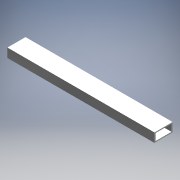
# Autodesk Inventor part: Extrusion Mid
Saved by Autodesk Inventor 2019.4 (Build 234330000, 330)
## iProperties
Created: 2020-01-07
Part Number: Extrusion Mid
Material: Aluminum 6061
Document SubType Name: Modeling
Designer: Mark
Mass: 453.827 g
Surface Area: 1128.84 cm^2
Volume: 168.084 cm^3
Density: 2.7 g/cm^3
Appearance: Aluminum - Flat
Author: Mark
Autodesk Inventor part; units mm, degrees
ref_plane "YZ Plane" through (0, 0, 0) normal (1, 0, 0) x (0, 1, 0)
ref_plane "XZ Plane" through (0, 0, 0) normal (0, 1, 0) x (-1, 0, 0)
ref_plane "XY Plane" through (0, 0, 0) normal (0, 0, 1) x (1, 0, 0)
sketch "Sketch1" plane through (0, 0, 0) normal (1, 0, 0) x (0, 1, 0)
  line L0 (-12.5, 25) -> (12.5, 25)
  line L1 (12.5, 25) -> (12.5, -25)
  line L2 (12.5, -25) -> (-12.5, -25)
  line L3 (-12.5, -25) -> (-12.5, 25)
  line L4 (-12.5, 25) -> (12.5, -25) construction
  line L5 (12.5, 25) -> (-12.5, -25) construction
  line L6 (-9.5, 22) -> (9.5, 22)
  line L7 (9.5, 22) -> (9.5, -22)
  line L8 (9.5, -22) -> (-9.5, -22)
  line L9 (-9.5, -22) -> (-9.5, 22)
  line L10 (-9.5, 22) -> (9.5, -22) construction
  line L11 (9.5, 22) -> (-9.5, -22) construction
  point P0 (0, 0)
  dimension "d0" = 25
  dimension "d1" = 50
  dimension "d2" = 19
  dimension "d3" = 44
  constraints: 24 end point, 4 midpoint, 4 parallel, 2 horizontal, 2 perpendicular
  measures "d0" distance of L1.end L2.end
  measures "d1" distance of L0.end L1.end
  measures "d2" distance of L7.end L8.end
  measures "d3" distance of L6.end L7.end
extrude "Extrusion1" add sketch "Sketch1" along normal blind 406
body "Solid1"
